# Autodesk Inventor part: 3WP
Saved by Autodesk Inventor 2013 (Build 170138000, 138)
## iProperties
Created: 2013-01-27
Part Number: 3WP
Material: Generic
Document SubType Name: Modeling
Designer: davidgitz
Density: 1 g/cm^3
Author: davidgitz
Autodesk Inventor part; units mm, degrees
ref_plane "YZ Plane" through (0, 0, 0) normal (1, 0, 0) x (0, 1, 0)
ref_plane "XZ Plane" through (0, 0, 0) normal (0, 1, 0) x (-1, 0, 0)
ref_plane "XY Plane" through (0, 0, 0) normal (0, 0, 1) x (1, 0, 0)
sketch "3, 3WP_3" plane through (0, 0, 0) normal (0, 0, 1) x (1, 0, 0)
  line L0 (-1.27, 1.27) -> (-1.27, -6.35)
  line L1 (-1.27, -6.35) -> (1.27, -6.35)
  line L2 (1.27, -6.35) -> (1.27, 1.27)
  line L3 (1.27, 1.27) -> (-1.27, 1.27)
  constraints: 8 end point
extrude "Extrusion1" add sketch "3, 3WP_3" along normal blind 3
body "Solid1"
